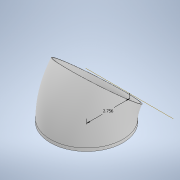
# Autodesk Inventor part: Fan_Part3
Saved by Autodesk Inventor 2020 (Build 240168000, 168)
## iProperties
Created: 2020-05-28
Part Number: Fan_Part3
Material: Generic
Document SubType Name: Modeling
Designer: maple
Density: 1 g/cm^3
Appearance: Default
Author: maple
Autodesk Inventor part; units mm, degrees
ref_plane "XZ Plane" through (0, 0, 0) normal (0, 1, 0) x (-1, 0, 0)
ref_plane "XY Plane" through (0, 0, 0) normal (0, 0, 1) x (1, 0, 0)
sketch "Sketch1" plane through (0, 0, 0) normal (0, 1, 0) x (-1, 0, 0)
  circle A0 centre (0, 0) radius 57.5
  line L0 (0, 57.5) -> (0, 59)
  circle A1 centre (0, 0) radius 59
  line L1 (82.6, -70) -> (-82.6, -70) projected
  dimension "d0" = 115
  dimension "d1" = 1.5
  constraints: 2 coincident, 2 end point, 2 vertical alignment, 1 vertical, 4 other
  measures "d1" distance of L0.start L0.end
sketch "Sketch2" plane through (0, 0, 0) normal (1, 0, 0) x (0, 1, 0)
  line L0 (0, 0) -> (0, -70)
  dimension "d2" = 70
  constraints: 2 end point, 1 vertical
  measures "d2" distance of L0.start L0.end
revolve "Revolution1" add sketch "Sketch1" angle 40 about axis through (0, 0, -70) along (-1, 0, 0)
sketch "Sketch3" plane through (0, 0, 0) normal (0, -1, 0) x (1, 0, 0)
  circle A0 centre (0, 0) radius 57.5
  circle A1 centre (0, 0) radius 59
  constraints: 2 centre point, 2 coincident
extrude "Extrusion1" add sketch "Sketch3" along normal blind 5
body "Solid1"
